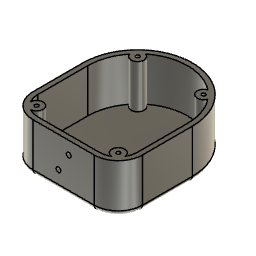
Microscope illuminator (Autodesk Fusion 360 design; units mm, degrees)
Autodesk Fusion 360 part; units mm, degrees
note: some values were not read from the file. Set by a fixed rule: which face or edge a step refers to.
sketch "Sketch1" plane through (0, 0, 0) normal (0, 0, 1) x (1, 0, 0)
  circle A0 centre (0, 0) radius 25.2
  line L0 (-34, 0) -> (0, 0) construction
  line L1 (34, 0) -> (0, 0) construction
  line L2 (-10, 21) -> (10, 21) construction
  line L3 (10, 21) -> (10, -39) construction
  line L4 (10, -39) -> (-10, -39) construction
  line L5 (-10, -39) -> (-10, 21) construction
  line L6 (0, -39) -> (0, 0) construction
  circle A1 centre (0, 0) radius 5 construction
  arc A2 (34, 0) -> (-34, 0) centre (0, 0) ccw
  line L7 (-34, 0) -> (-34, -46)
  line L8 (34, 0) -> (34, -46)
  line L9 (34, -46) -> (-34, -46)
  circle A3 centre (0, 0) radius 22.2
  dimension "d3" = 50.4
  dimension "d4" = 68
  dimension "d5" = 60
  dimension "d6" = 20
  dimension "d7" = 39
  dimension "d8" = 10
  dimension "d9" = 3
  dimension "d11" = 46
  constraint concentric A0 A2
  constraint coincident A0.centre L0.end
  constraint horizontal L0
  constraint horizontal L2
  constraint vertical L3
  constraint horizontal L4
  constraint vertical L5
  constraint midpoint L4 L6.start
  constraint perpendicular L4 L6
  constraint tangent A2 L7
  constraint tangent A2 L8
  constraint perpendicular L1 L8
  constraint horizontal L9
  constraint concentric A2 A3
  measures "d3" diameter of A0
  measures "d4" diameter of A2
  measures "d5" distance of L2.start L4.end
  measures "d6" distance of L2.start L2.end
  measures "d7" distance of L6.start A0.centre
  measures "d8" diameter of A1
  measures "d9" distance of A0 A3
  measures "d11" distance of L0.start L7.end
extrude "Extrude1" add sketch "Sketch1" along normal blind 10 contours A0 makes body 1
extrude "Extrude2" add sketch "Sketch1" along normal blind 3 contours A2 L7 L8 L9 bodies 1
sketch "Sketch2" plane through (0, 0, 0) normal (1, 0, 0) x (0, 1, 0)
  line L0 (0, 10) -> (0, 3) construction
  circle A0 centre (0, 6.5) radius 1
  point P0 (0, 3)
  point P1 (0, 10)
  dimension "d16" = 2
  constraint coincident P1 L0.start
  constraint coincident P0 L0.end
  constraint midpoint L0 A0.centre
  measures "d16" diameter of A0
extrude "Extrude3" cut sketch "Sketch2" along normal through all and the other way through all bodies 1
fillet "Fillet1" radius 15 2 edges at (-34, -46, 1.5) (34, -46, 1.5) on bodies 1
sketch "Sketch3" plane through (0, 0, 0) normal (0, 0, 1) x (1, 0, 0)
  arc A0 (19, -46) -> (34, -31) centre (19, -31) ccw
  line L0 (19, -46) -> (-19, -46)
  arc A1 (-34, -31) -> (-19, -46) centre (-19, -31) ccw
  line L1 (-34, -31) -> (-34, 0)
  arc A2 (34, 0) -> (-34, 0) centre (0, 0) ccw
  line L2 (34, 0) -> (34, -31)
  circle A3 centre (0, 0) radius 22.2
extrude "Extrude4" add sketch "Sketch3" against normal blind 30 separate body contours A0 L0 A1 L1 A2 L2 | A3 makes body 2
fillet "Fillet2" radius 3 6 edges at (29.6066, -41.6066, -30) (0, -46, -30) (-29.6066, -41.6066, -30) (-34, -15.5, -30) (0, 34, -30) (34, -15.5, -30) on bodies 2
shell "Shell1" thickness 3 removed faces 1 at (6.3333, -15.3333, 0) on bodies 2
sketch "Sketch4" plane through (0, -46, 0) normal (0, -1, 0) x (1, 0, 0)
  line L0 (-19, -27) -> (19, -27)
  line L1 (19, -27) -> (19, 0)
  line L2 (19, 0) -> (-19, 0)
  line L3 (-19, 0) -> (-19, -27)
  line L4 (0, 0) -> (0, -27) construction
  circle A0 centre (0, -13.5) radius 6.3791 construction
  line L5 (0, -13.5) -> (3.1896, -7.9755) construction
  circle A1 centre (3.1896, -7.9755) radius 1.5
  line L6 (3.1896, -7.9755) -> (-3.1896, -19.0245) construction
  circle A2 centre (-3.1896, -19.0245) radius 1.5
  circle A3 centre (-3.1896, -19.0245) radius 4
  circle A4 centre (3.1896, -7.9755) radius 4
  dimension "d26" = 30
  dimension "d27" = 3
  dimension "d28" = 3
  dimension "d31" = 2.5
  dimension "d32" = 2.5
  constraint coincident L4.start origin
  constraint midpoint L0 L4.end
  constraint midpoint L4 A0.centre
  constraint coincident A0.centre L5.start
  constraint coincident A0 L5.end
  constraint coincident L5.end A1.centre
  constraint coincident A0 L6.end
  constraint parallel L5 L6
  constraint coincident L6.end A2.centre
  constraint concentric A2 A3
  measures "d26" angle of L4 L5
  measures "d27" diameter of A1
  measures "d28" diameter of A2
  measures "d31" distance of A1 A4
  measures "d32" distance of A2 A3
extrude "Extrude5" cut sketch "Sketch4" against normal up to surface (3 mm away) contours A1 | A2 bodies 2
extrude "Extrude6" add sketch "Sketch4" against normal blind 3 from surface at -3 contours A3 | A4 bodies 2
ref_plane "WorkPlane1" through (3.1896, -40.8716, -11.9755) normal (0, 0, -1) x (1, 0, 0)
sketch "Sketch5" plane through (0, 0, -11.9755) normal (0, 0, -1) x (-1, 0, 0)
  line L0 (0.8104, -40) -> (-7.1896, -40)
  line L1 (-0.8104, -43) -> (7.1896, -43)
  line L2 (-7.1896, -43) -> (0.8104, -43)
  line L3 (19, -43) -> (-19, -43)
  line L4 (-3.1896, -40) -> (-3.1896, -43) construction
  line L5 (-3.6896, -43) -> (-3.6896, -40)
  line L6 (-2.6896, -43) -> (-2.6896, -40)
  line L7 (-19, -43) -> (19, -43)
  dimension "d37" = 1
  constraint midpoint L0 L4.start
  constraint midpoint L2 L4.end
  constraint coincident L0 L5.end
  constraint perpendicular L0 L5
  constraint symmetric L4 L5.start L6.start
  constraint symmetric L4 L5.end L6.end
  measures "d37" distance of L5 L6
extrude "Extrude7" add sketch "Sketch5" against normal blind 0.521 separate body makes body 3
move_face "OffsetFaces1" offset 3 1 faces at (3.3562, -41, -11.9755) on bodies 3
chamfer "Chamfer1" distance 3 angle 45 1 edges at (3.1896, -40, -14.9755) on bodies 3
copy_body "CopyPasteBodies1" bodies 3 makes body 4
move_body "Move1" bodies 4 to x (1, 0, 0) y (0, 1, 0) z (0, 0, 1) at (-6.3662, 0, -11.055)
combine "Combine1" operation add target body 2 tool bodies 3 4
sketch "Sketch6" plane through (0, 0, -27) normal (0, 0, 1) x (-1, 0, 0)
  line L0 (-20, 0) -> (-2.5, 0)
  line L1 (0, 0) -> (0, 23.7257) construction
  line L2 (0, 0) -> (-24.0416, -24.0416) construction
  circle A0 centre (-20.5061, -20.5061) radius 4
  arc A1 (-34, 0) -> (34, 0) centre (0, 0) ccw
  line L3 (-22.5355, 34.5355) -> (-29.6066, 41.6066) construction
  line L4 (-19, 46) -> (19, 46)
  arc A2 (-19, 46) -> (-34, 31) centre (-19, 31) ccw
  circle A3 centre (-25.364, 37.364) radius 4
  circle A4 centre (-20.5061, -20.5061) radius 1.15
  circle A5 centre (-25.364, 37.364) radius 1.15
  circle A6 centre (20.5061, -20.5061) radius 4
  circle A7 centre (20.5061, -20.5061) radius 1.15
  circle A8 centre (25.364, 37.364) radius 4
  circle A9 centre (25.364, 37.364) radius 1.15
  line L5 (31, 0) -> (31, 31)
  arc A10 (31, 31) -> (19, 43) centre (19, 31) ccw
  line L6 (19, 43) -> (-19, 43)
  arc A11 (-19, 43) -> (-31, 31) centre (-19, 31) ccw
  line L7 (-31, 31) -> (-31, 0)
  arc A12 (-31, 0) -> (31, 0) centre (0, 0) ccw
  dimension "d48" = 45
  dimension "d49" = 8
  dimension "d50" = 5
  dimension "d51" = 45
  dimension "d52" = 8
  dimension "d53" = 6
  dimension "d54" = 2.3
  dimension "d56" = 2.3
  constraint perpendicular L0 L1
  constraint coincident L1.start L2.start
  constraint coincident L2 A0.centre
  constraint coincident L2.end A1
  constraint midpoint L3.end A2
  constraint coincident L3 A3.centre
  constraint concentric A0 A4
  constraint concentric A3 A5
  constraint symmetric L1 A0 A6
  constraint symmetric L1 A3 A8
  constraint symmetric L1 A4 A7
  constraint symmetric L1 A5 A9
  measures "d48" angle of L0 L2
  measures "d49" diameter of A0
  measures "d50" distance of L2.end A0.centre
  measures "d51" angle of L3 L4
  measures "d52" diameter of A3
  measures "d53" distance of L3.end A3.centre
  measures "d54" diameter of A4
  measures "d56" diameter of A5
extrude "Extrude9" add sketch "Sketch6" along normal blind 27 contours A0 A12 | A0 A12 | A6 A12 | A6 A12 | A3 A11 | A3 A11 | A8 A10 | A8 A10 bodies 2
sketch "Sketch7" plane through (0, 0, 3) normal (0, 0, 1) x (-1, 0, 0)
  arc A0 (-19, 46) -> (-34, 31) centre (-19, 31) ccw
  line L0 (-34, 31) -> (-34, 0)
  arc A1 (-34, 0) -> (34, 0) centre (0, 0) ccw
  line L1 (34, 0) -> (34, 31)
  arc A2 (34, 31) -> (19, 46) centre (19, 31) ccw
  line L2 (19, 46) -> (-19, 46)
  circle A3 centre (0, 0) radius 25.2
  point P0 (25.364, 37.364)
  point P1 (-25.364, 37.364)
  point P2 (20.5061, -20.5061)
  point P3 (-20.5061, -20.5061)
hole "Hole1" at (-25.364, -37.364, 3) at (25.364, -37.364, 3) at (-20.5061, 20.5061, 3) at (20.5061, 20.5061, 3) direction (0, 0, -1) diameter 2.9 depth 5.3 tip angle 118 countersink diameter 5.2 countersink angle 90 bodies 1
hidden bodies 1
equation "d31 = d32"
equation "d52 = d49"
